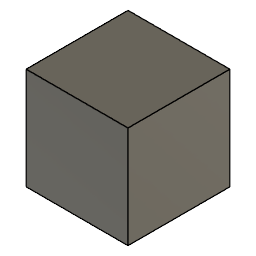
cubeplayerpiece2 (Autodesk Fusion 360 archive; units mm, degrees)
design "cube2"
Autodesk Fusion 360 part; units mm, degrees
sketch "Sketch1" plane through (0, 0, 0) normal (0, 0, 1) x (1, 0, 0)
  line L0 (0, 0) -> (0, 22.86)
  line L1 (0, 22.86) -> (22.86, 22.86)
  line L2 (22.86, 22.86) -> (22.86, 0)
  line L3 (22.86, 0) -> (0, 0)
  dimension "d1" = 22.86
  dimension "d2" = 22.86
  constraint coincident L0.start L3.end
  constraint vertical L0
  constraint perpendicular L0 L1
  constraint perpendicular L1 L2
  constraint perpendicular L0 L3
  measures "d1" distance of L0.start L0.end
  measures "d2" distance of L0.end L1.end
extrude "Extrude1" add sketch "Sketch1" along normal blind 22.86

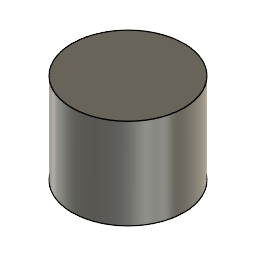
design "playerbase2"
Autodesk Fusion 360 part; units mm, degrees
sketch "Sketch1" plane through (0, 0, 0) normal (0, 0, 1) x (1, 0, 0)
  circle A0 centre (0, 0) radius 2.3495
  dimension "d1" = 4.699
  constraint coincident A0.centre origin
  measures "d1" diameter of A0
extrude "Extrude1" add sketch "Sketch1" along normal blind 3.81
